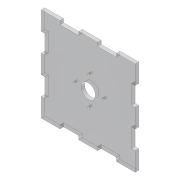
# Autodesk Inventor part: M01 - Base Top
Saved by Autodesk Inventor 2016 (Build 200138000, 138)
## iProperties
Created: 2016-12-26
Part Number: M01 - Base Top
Material: Polycarbonate, Clear
Document SubType Name: Modeling
Designer: Fernando
Stock Number: 0
Mass: 389.272 g
Surface Area: 900.964 cm^2
Volume: 324.393 cm^3
Density: 1.2 g/cm^3
Appearance: Polycarbonate - Clear
SurfaceArea_m2: .09
Author: Fernando
Autodesk Inventor part; units mm, degrees
ref_plane "YZ Plane" through (0, 0, 0) normal (1, 0, 0) x (0, 1, 0)
ref_plane "XZ Plane" through (0, 0, 0) normal (0, 1, 0) x (-1, 0, 0)
ref_plane "XY Plane" through (0, 0, 0) normal (0, 0, 1) x (1, 0, 0)
sketch "Sketch2" plane through (0, 0, 0) normal (0, 1, 0) x (-1, 0, 0)
  line L0 (-105, 105) -> (105, 105)
  line L1 (105, 105) -> (105, -105)
  line L2 (105, -105) -> (-105, -105)
  line L3 (-105, -105) -> (-105, 105)
  line L4 (-105, 105) -> (105, -105) construction
  line L5 (105, 105) -> (-105, -105) construction
  circle A0 centre (0, 0) radius 15.95
  dimension "d11" = 210
  dimension "d12" = 210
  dimension "d13" = 31.9
  constraints: 12 end point, 2 midpoint, 2 parallel, 1 centre point, 1 coincident, 1 horizontal, 1 perpendicular
  measures "d11" distance of L1.end L2.end
  measures "d12" distance of L2.end L0.start
  measures "d13" diameter of A0
extrude "Extrusion2" add sketch "Sketch2" along normal blind 8
sketch "Sketch3" plane through (0, 0, 0) normal (0, -1, 0) x (1, 0, 0)
  point P0 (0, 0)
  point P1 (32, 0)
  dimension "d16" = 32
  constraints: 1 horizontal alignment
  measures "d16" distance of point (32, 0) point (0, 0)
hole "Hole1" at (32, 0, 0) direction (0, 1, 0) diameter 4.5 depth 8 tip angle 118
pattern_circular "Circular Pattern1" count 4 over 360 about axis through (0, 0, 0) along (0, 1, 0) of "Hole1"
sketch "Sketch4" plane through (0, 0, 0) normal (0, -1, 0) x (1, 0, 0)
  circle A0 centre (0, 32) radius 2.25 projected
  circle A1 centre (-32, 0) radius 2.25 projected
  circle A2 centre (0, -32) radius 2.25 projected
  circle A3 centre (32, 0) radius 2.25 projected
  circle A4 centre (0, 0) radius 15.95 projected
  line L0 (105, 105) -> (-105, 105) projected
  line L1 (-105, 105) -> (-105, -105) projected
  line L2 (-105, -105) -> (105, -105) projected
  line L3 (105, -105) -> (105, 105) projected
  line L4 (-105, -63) -> (-97, -63)
  line L5 (-97, -63) -> (-97, -21)
  line L6 (-97, -21) -> (-105, -21)
  line L7 (-105, -21) -> (-105, -63)
  line L8 (-105, 21) -> (-97, 21)
  line L9 (-97, 21) -> (-97, 63)
  line L10 (-97, 63) -> (-105, 63)
  line L11 (-105, 63) -> (-105, 21)
  line L12 (-97, -21) -> (-97, 21) construction
  line L13 (-97, 63) -> (-97, 105) construction
  line L14 (-97, -63) -> (-97, -105)
  dimension "d27" = 8
  constraints: 22 end point, 6 point on line, 4 collinear, 4 parallel, 3 perpendicular, 2 horizontal, 1 vertical
  measures "d27" distance of L4.start L4.end
extrude "Extrusion3" cut sketch "Sketch4" against normal through all contours L10 L9 L8 L1 | L4 L1 L6 L5
sketch "Sketch5" plane through (0, 0, 0) normal (0, -1, 0) x (1, 0, 0)
  line L0 (-97, 21) -> (-105, 21) projected
  line L1 (-105, 21) -> (-105, -21) projected
  line L2 (-105, -21) -> (-97, -21) projected
  line L3 (-97, -21) -> (-97, -63) projected
  line L4 (-97, -63) -> (-105, -63) projected
  line L5 (-105, -63) -> (-105, -105) projected
  line L6 (-105, -105) -> (105, -105) projected
  line L7 (105, -105) -> (105, 105) projected
  line L8 (105, 105) -> (-105, 105) projected
  line L9 (-105, 105) -> (-105, 63) projected
  line L10 (-105, 63) -> (-97, 63) projected
  line L11 (-97, 63) -> (-97, 21) projected
  circle A0 centre (0, 32) radius 2.25 projected
  circle A1 centre (-32, 0) radius 2.25 projected
  circle A2 centre (0, -32) radius 2.25 projected
  circle A3 centre (32, 0) radius 2.25 projected
  circle A4 centre (0, 0) radius 15.95 projected
  line L12 (63, -105) -> (21, -105)
  line L13 (21, -105) -> (21, -97)
  line L14 (21, -97) -> (63, -97)
  line L15 (63, -97) -> (63, -105)
  line L16 (-21, -105) -> (-63, -105)
  line L17 (-63, -105) -> (-63, -97)
  line L18 (-63, -97) -> (-21, -97)
  line L19 (-21, -97) -> (-21, -105)
  line L20 (63, -97) -> (105, -97) construction
  line L21 (21, -97) -> (-21, -97) construction
  line L22 (-63, -97) -> (-105, -97) construction
  dimension "d31" = 8
  constraints: 22 end point, 6 point on line, 5 equal length, 4 collinear, 3 horizontal, 2 perpendicular
  measures "d31" distance of L12.end L13.end
extrude "Extrusion4" cut sketch "Sketch5" against normal through all contours L6 L13 L14 L15 | L17 L18 L19 L6
mirror "Mirror1" about plane through (0, 0, 0) normal (1, 0, 0) of "Extrusion3"
mirror "Mirror2" about plane through (0, 0, 0) normal (0, 0, 1) of "Extrusion4"
equation "\"d11\" = d12"
body "Solid2"
